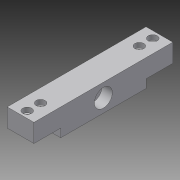
# Autodesk Inventor part: hph_C_001
Saved by Autodesk Inventor 2014 (Build 180170000, 170)
## iProperties
Created: 2014-03-22
Part Number: hph_C_001
Material: Generic
Document SubType Name: Modeling
Designer: stephenholtz
Density: 1 g/cm^3
Appearance: Default
Mass: 10.318 g
Surface Area: 53.3752 cm^2
Volume: 10.318 cm^3
Description: CNC 302 Stainless Steel
Author: stephenholtz
Revision Number: 1
Autodesk Inventor part; units mm, degrees
ref_plane "YZ Plane" through (0, 0, 0) normal (1, 0, 0) x (0, 1, 0)
ref_plane "XZ Plane" through (0, 0, 0) normal (0, 1, 0) x (-1, 0, 0)
sketch "Sketch2" plane through (0, 0, 0) normal (0, 0, 1) x (1, 0, 0)
  line L0 (-42.8625, -8.255) -> (42.8625, -8.255)
  line L1 (42.8625, -8.255) -> (42.8625, 8.255)
  line L2 (42.8625, 8.255) -> (-42.8625, 8.255)
  line L3 (-42.8625, 8.255) -> (-42.8625, -8.255)
  line L4 (-42.8625, -8.255) -> (42.8625, 8.255) construction
  line L5 (42.8625, -8.255) -> (-42.8625, 8.255) construction
  point P0 (0, 0)
  dimension "bar_length" = 85.725
  dimension "bar_width" = 16.51
  constraints: 12 end point, 2 midpoint, 2 parallel, 1 horizontal, 1 perpendicular
  measures "bar_length" distance of L1.end L2.end
  measures "bar_width" distance of L2.end L0.start
extrude "Extrusion1" add sketch "Sketch2" along normal blind 16.51
ref_plane "Work Plane1" through (0, -8.255, 0) normal (1, 0, 0) x (0, 0, -1)
sketch "Sketch5" plane through (0, 0, 0) normal (0, 0, -1) x (-1, 0, 0)
  line L0 (42.8625, -8.255) -> (-42.8625, -8.255) construction
  line L1 (42.8625, 8.255) -> (42.8625, -8.255) construction
  line L2 (-42.8625, 8.255) -> (42.8625, 8.255) construction
  line L3 (-42.8625, -8.255) -> (-42.8625, 8.255) construction
  line L4 (-42.8625, -8.255) -> (-26.3525, -8.255) construction
  line L5 (-26.3525, -8.255) -> (-26.3525, 8.255) construction
  line L6 (-26.3525, 8.255) -> (-42.8625, 8.255) construction
  line L7 (-42.8625, 8.255) -> (-42.8625, -8.255) construction
  line L8 (-34.6075, -8.255) -> (-34.6075, 8.255) construction
  line L9 (-38.735, -8.255) -> (-38.735, 8.255) construction
  line L10 (-30.48, -8.255) -> (-30.48, 8.255) construction
  line L11 (-34.6075, -8.255) -> (-34.6075, 8.255) construction
  point P0 (0, 0)
  point P1 (-30.48, 0)
  point P2 (-38.735, 0)
  dimension "d10" = 16.51
  dimension "d11" = 16.51
  dimension "d14" = 4.1275
  dimension "d17" = 4.1275
  constraints: 16 end point, 4 midpoint, 3 horizontal, 2 parallel, 1 perpendicular, 1 point on line, 9 other
  measures "d10" distance of L0.end L4.end
  measures "d11" distance of L0.end L2.start
  measures "d14" distance of L8.start L9.start
  measures "d17" distance of L8.start L10.start
hole "Hole1" at (30.48, 0, 0) at (38.735, 0, 0) direction (0, 0, 1) diameter 3.4544 end through all counterbore diameter 5.5626 counterbore depth 3.048
sketch "Sketch4" plane through (0, 0, 16.51) normal (0, 0, 1) x (1, 0, 0)
  line L0 (-42.8625, -8.255) -> (42.8625, -8.255) construction
  line L1 (42.8625, -8.255) -> (42.8625, 8.255) construction
  line L2 (42.8625, 8.255) -> (-42.8625, 8.255) construction
  line L3 (-42.8625, 8.255) -> (-42.8625, -8.255) construction
  line L4 (42.8625, -8.255) -> (26.3525, -8.255)
  line L5 (26.3525, -8.255) -> (26.3525, 8.255)
  line L6 (26.3525, 8.255) -> (42.8625, 8.255)
  line L7 (42.8625, 8.255) -> (42.8625, -8.255)
  circle A0 centre (38.735, 0) radius 1.7272 projected
  point P0 (0, 0)
  dimension "d6" = 16.51
  dimension "d7" = 16.51
  constraints: 8 end point, 2 parallel, 1 horizontal, 1 perpendicular, 1 point on line
  measures "d6" distance of L0.end L4.end
  measures "d7" distance of L0.end L1.end
extrude "Extrusion2" cut sketch "Sketch4" against normal blind 5.207 contours L4 L5 L6 L7 | A0
mirror "Mirror2" about plane through (0, -8.255, 0) normal (1, 0, 0) of "Hole1", "Extrusion2"
sketch "Sketch7" plane through (-42.8625, -8.255, 0) normal (0, -1, 0) x (1, 0, 0)
  line L0 (0, 0) -> (85.725, 0) projected
  line L1 (85.725, 0) -> (85.725, 11.303) projected
  line L2 (16.51, 16.51) -> (69.215, 16.51) projected
  line L3 (0, 0) -> (0, 11.303) projected
  line L4 (55.5625, 8.255) -> (42.8625, 8.255)
  line L5 (0, 16.51) -> (85.725, 16.51) projected
  line L6 (42.8625, 8.255) -> (30.1625, 8.255)
  line L7 (85.725, 8.255) -> (0, 8.255) construction
  line L8 (42.8625, 0) -> (42.8625, 16.51) construction
  line L9 (16.51, 16.51) -> (16.51, 11.303) projected
  line L10 (16.51, 11.303) -> (0, 11.303) projected
  line L11 (85.725, 11.303) -> (69.215, 11.303) projected
  line L12 (69.215, 11.303) -> (69.215, 16.51) projected
  dimension "d48" = 12.7
  constraints: 8 end point, 2 collinear, 2 midpoint, 2 parallel, 2 point on line
  measures "d48" distance of L4.end L4.start
hole "Hole6" at (0, -8.255, 8.255) direction (0, 1, 0) diameter 6.7564 end through all counterbore diameter 11.1252 counterbore depth 6.35 clearance for "Socket Head Cap Screw" size "1/4" standard "Ansi Unified Screw Threads"
equation "\"d2\" = bar_width"
equation "\"d14\" = 0.5 * hole_spacing"
equation "\"d17\" = 0.5 * hole_spacing"
equation "\"hole_spacing\" = 8.255"
body "Solid1"
